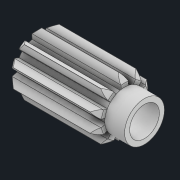
# Autodesk Inventor part: Steering Gear
Saved by Autodesk Inventor 2021 (Build 250183000, 183)
## iProperties
Created: 2020-10-15
Part Number: Steering Gear
Material: Generic
Document SubType Name: Modeling
Designer: Eugene Tang
Mass: 13.0101 g
Surface Area: 104.256 cm^2
Volume: 13.0101 cm^3
Density: 1 g/cm^3
Appearance: Default
ToothH: 5.620 mm
contact: 26.000 mm
rackteethprofileDepth: 2.411 mm
rackteethprofileLong: 3.683 mm
rackteethprofileShort: 2.480 mm
SteererGearPlane: 18.760 mm
GearLength: 45.000 mm
d1: 15.000 mm
Author: Eugene Tang
Autodesk Inventor part; units mm, degrees
ref_plane "YZ Plane" through (0, 0, 0) normal (1, 0, 0) x (0, 1, 0)
ref_plane "XZ Plane" through (0, 0, 0) normal (0, 1, 0) x (-1, 0, 0)
ref_plane "XY Plane" through (0, 0, 0) normal (0, 0, 1) x (1, 0, 0)
sketch "Sketch1" plane through (0, 0, 0) normal (1, 0, 0) x (0, 1, 0)
  circle A0 centre (0, 0) radius 11 construction
  circle A1 centre (0, 0) radius 7.5
  circle A2 centre (0, 0) radius 15
  line L0 (0, 0) -> (10.8109, -2.0308) construction
  line L1 (0, 0) -> (10.9093, 1.4093) construction
  line L2 (0, 0) -> (9.9399, 4.7115) construction
  line L3 (0, 0) -> (7.9975, 7.5525) construction
  line L4 (0, 0) -> (5.2722, 9.6542) construction
  line L5 (0, 0) -> (2.0308, 10.8109) construction
  line L6 (2.0308, 10.8109) -> (18.9428, 7.634) construction
  line L7 (5.2722, 9.6542) -> (17.3542, 3.0562) construction
  line L8 (7.9975, 7.5525) -> (15.0863, 0.0461) construction
  line L9 (9.9399, 4.7115) -> (12.8881, -1.5082) construction
  line L10 (10.9093, 1.4093) -> (10.8109, -2.0308) construction
  spline S0 degree 4 poles (10.8109, -2.0308) (13.448, -1.9078) (15.839, -0.0396) (18.3147, 3.5093) (18.9428, 7.634) knots 0 0 0 0 0 1 1 1 1 1 construction
  circle A3 centre (0, 0) radius 12 construction
  circle A4 centre (0, 0) radius 15.5 construction
  line L11 (0, 0) -> (15.3092, -2.4247) construction
  line L12 (-22.7177, 0) -> (27.8064, 0) construction
  circle A5 centre (0, 0) radius 9.38
  line L13 (11.8523, -1.8772) -> (-15, 0) construction
  circle A6 centre (0, 0) radius 13 construction
  dimension "d0" = 22
  dimension "d2" = 30
  dimension "d14" = 24
  dimension "d15" = 0.5
  dimension "d30" = 4
  dimension "d1" = 15
  dimension "angle" = 90
  dimension "d9" = 6.8831
  dimension "d10" = 10.3247
  dimension "d11" = 13.7662
  dimension "d13" = 17.2078
  dimension "d16" = 9
  dimension "SteererGearPlane" = 18.76
  dimension "ToothH" = 5.62
  dimension "d31" = 2
  dimension "contact" = 26
  constraints: 26 end point, 7 coincident, 3 centre point, 1 concentric, 1 horizontal alignment, 1 point on line, 39 other
  measures "d1" diameter of A1
  measures "d9" distance of L2.end L9.end
  measures "d10" distance of L3.end L8.end
  measures "d11" distance of L4.end L7.end
  measures "d13" distance of L5.end L6.end
  measures "d16" angle to the sketch x axis of L11
  measures "SteererGearPlane" diameter of A5
  measures "contact" diameter of A6
sketch "Sketch2" plane through (0, 0, 0) normal (1, 0, 0) x (0, 1, 0)
  circle A0 centre (0, 0) radius 12 construction
  line L0 (10.9093, 1.4093) -> (10.8109, -2.0308) construction
  line L1 (9.9399, 4.7115) -> (12.8881, -1.5082) construction
  line L2 (7.9975, 7.5525) -> (15.0863, 0.0461) construction
  line L3 (5.2722, 9.6542) -> (17.3542, 3.0562) construction
  line L4 (2.0308, 10.8109) -> (18.9428, 7.634) construction
  circle A1 centre (0, 0) radius 7.5 projected
  circle A2 centre (0, 0) radius 9.38 projected
  circle A3 centre (0, 0) radius 15 projected
  line L5 (11.8523, -1.8772) -> (-15, 0) construction
  spline S0 degree 4 poles (10.8109, -2.0308) (13.448, -1.9078) (15.839, -0.0396) (18.3147, 3.5093) (18.9428, 7.634) knots 0 0 0 0 0 1 1 1 1 1
  line L6 (11.8523, -1.8772) -> (9.2258, -1.6936)
  line L7 (-28.8241, 0) -> (28.8241, 0) construction
  spline S1 degree 4 poles (10.8109, 2.0308) (13.448, 1.9078) (15.839, 0.0396) (18.3147, -3.5093) (18.9428, -7.634) knots 0 0 0 0 0 1 1 1 1 1
  line L8 (11.8523, 1.8772) -> (9.2258, 1.6936)
  spline S2 degree 4 poles (9.9399, 4.7115) (12.0011, 6.3611) (12.8373, 9.2779) (12.7542, 13.6042) (10.8379, 17.3103) knots 0 0 0 0 0 1 1 1 1 1
  spline S3 degree 4 poles (7.5525, 7.9975) (9.7583, 9.448) (12.7908, 9.3419) (16.8796, 7.9261) (19.8122, 4.9583) knots 0 0 0 0 0 1 1 1 1 1
  line L9 (8.4853, 8.4853) -> (6.4684, 6.793)
  line L10 (10.6921, 5.4479) -> (8.4593, 4.0527)
  spline S4 degree 4 poles (5.2722, 9.6542) (5.9701, 12.2003) (4.9321, 15.0516) (2.3221, 18.5028) (-1.4067, 20.3747) knots 0 0 0 0 0 1 1 1 1 1
  spline S5 degree 4 poles (1.4093, 10.9093) (2.3413, 13.3794) (4.8569, 15.076) (8.9971, 16.3339) (13.114, 15.6566) knots 0 0 0 0 0 1 1 1 1 1
  line L11 (1.8772, 11.8523) -> (1.2402, 9.2976)
  line L12 (5.4479, 10.6921) -> (4.4617, 8.2509)
  spline S6 degree 4 poles (-1.4093, 10.9093) (-2.3413, 13.3794) (-4.8569, 15.076) (-8.9971, 16.3339) (-13.114, 15.6566) knots 0 0 0 0 0 1 1 1 1 1
  spline S7 degree 4 poles (-5.2722, 9.6542) (-5.9701, 12.2003) (-4.9321, 15.0516) (-2.3221, 18.5028) (1.4067, 20.3747) knots 0 0 0 0 0 1 1 1 1 1
  line L13 (-5.4479, 10.6921) -> (-4.4617, 8.2509)
  line L14 (-1.8772, 11.8523) -> (-1.2402, 9.2976)
  spline S8 degree 4 poles (-7.5525, 7.9975) (-9.7583, 9.448) (-12.7908, 9.3419) (-16.8796, 7.9261) (-19.8122, 4.9583) knots 0 0 0 0 0 1 1 1 1 1
  spline S9 degree 4 poles (-9.9399, 4.7115) (-12.0011, 6.3611) (-12.8373, 9.2779) (-12.7542, 13.6042) (-10.8379, 17.3103) knots 0 0 0 0 0 1 1 1 1 1
  line L15 (-10.6921, 5.4479) -> (-8.4593, 4.0527)
  line L16 (-8.4853, 8.4853) -> (-6.4684, 6.793)
  spline S10 degree 4 poles (-10.8109, 2.0308) (-13.448, 1.9078) (-15.839, 0.0396) (-18.3147, -3.5093) (-18.9428, -7.634) knots 0 0 0 0 0 1 1 1 1 1
  spline S11 degree 4 poles (-10.8109, -2.0308) (-13.448, -1.9078) (-15.839, -0.0396) (-18.3147, 3.5093) (-18.9428, 7.634) knots 0 0 0 0 0 1 1 1 1 1
  line L17 (-11.8523, -1.8772) -> (-9.2258, -1.6936)
  line L18 (-11.8523, 1.8772) -> (-9.2258, 1.6936)
  spline S12 degree 4 poles (-9.9399, -4.7115) (-12.0011, -6.3611) (-12.8373, -9.2779) (-12.7542, -13.6042) (-10.8379, -17.3103) knots 0 0 0 0 0 1 1 1 1 1
  spline S13 degree 4 poles (-7.5525, -7.9975) (-9.7583, -9.448) (-12.7908, -9.3419) (-16.8796, -7.9261) (-19.8122, -4.9583) knots 0 0 0 0 0 1 1 1 1 1
  line L19 (-8.4853, -8.4853) -> (-6.4684, -6.793)
  line L20 (-10.6921, -5.4479) -> (-8.4593, -4.0527)
  spline S14 degree 4 poles (-5.2722, -9.6542) (-5.9701, -12.2003) (-4.9321, -15.0516) (-2.3221, -18.5028) (1.4067, -20.3747) knots 0 0 0 0 0 1 1 1 1 1
  spline S15 degree 4 poles (-1.4093, -10.9093) (-2.3413, -13.3794) (-4.8569, -15.076) (-8.9971, -16.3339) (-13.114, -15.6566) knots 0 0 0 0 0 1 1 1 1 1
  line L21 (-1.8772, -11.8523) -> (-1.2402, -9.2976)
  line L22 (-5.4479, -10.6921) -> (-4.4617, -8.2509)
  spline S16 degree 4 poles (1.4093, -10.9093) (2.3413, -13.3794) (4.8569, -15.076) (8.9971, -16.3339) (13.114, -15.6566) knots 0 0 0 0 0 1 1 1 1 1
  spline S17 degree 4 poles (5.2722, -9.6542) (5.9701, -12.2003) (4.9321, -15.0516) (2.3221, -18.5028) (-1.4067, -20.3747) knots 0 0 0 0 0 1 1 1 1 1
  line L23 (5.4479, -10.6921) -> (4.4617, -8.2509)
  line L24 (1.8772, -11.8523) -> (1.2402, -9.2976)
  spline S18 degree 4 poles (7.5525, -7.9975) (9.7583, -9.448) (12.7908, -9.3419) (16.8796, -7.9261) (19.8122, -4.9583) knots 0 0 0 0 0 1 1 1 1 1
  spline S19 degree 4 poles (9.9399, -4.7115) (12.0011, -6.3611) (12.8373, -9.2779) (12.7542, -13.6042) (10.8379, -17.3103) knots 0 0 0 0 0 1 1 1 1 1
  line L25 (10.6921, -5.4479) -> (8.4593, -4.0527)
  line L26 (8.4853, -8.4853) -> (6.4684, -6.793)
  arc A4 (-9.2258, -1.6936) -> (-8.4593, -4.0527) centre (0, 0) ccw
  arc A5 (-6.4684, -6.793) -> (-4.4617, -8.2509) centre (0, 0) ccw
  arc A6 (-1.2402, -9.2976) -> (1.2402, -9.2976) centre (0, 0) ccw
  arc A7 (4.4617, -8.2509) -> (6.4684, -6.793) centre (0, 0) ccw
  arc A8 (8.4593, -4.0527) -> (9.2258, -1.6936) centre (0, 0) ccw
  arc A9 (9.2258, 1.6936) -> (8.4593, 4.0527) centre (0, 0) ccw
  arc A10 (6.4684, 6.793) -> (4.4617, 8.2509) centre (0, 0) ccw
  arc A11 (1.2402, 9.2976) -> (-1.2402, 9.2976) centre (0, 0) ccw
  arc A12 (-4.4617, 8.2509) -> (-6.4684, 6.793) centre (0, 0) ccw
  arc A13 (-8.4593, 4.0527) -> (-9.2258, 1.6936) centre (0, 0) ccw
  line L27 (1.2402, -9.2976) -> (-1.2402, -9.2976) construction
  line L28 (-0.4196, -9.2976) -> (-0.4196, -11.7086) construction
  line L29 (1.8414, -11.7086) -> (-1.8414, -11.7086) construction
  point P0 (12.8881, 1.5082)
  point P1 (15.0863, -0.0461)
  point P2 (17.3542, -3.0562)
  point P3 (12.178, 8.9048)
  point P4 (12.2434, 12.6731)
  point P5 (11.3132, 6.3552)
  point P6 (12.2322, 8.8303)
  point P7 (15.8363, 7.728)
  point P8 (9.5402, 8.7956)
  point P9 (4.6181, 14.3622)
  point P10 (2.4561, 17.4493)
  point P11 (5.4171, 11.7912)
  point P12 (4.7057, 14.3337)
  point P13 (8.2694, 15.5604)
  point P14 (2.5482, 12.7234)
  point P15 (-4.7057, 14.3337)
  point P16 (-8.2694, 15.5604)
  point P17 (-2.5482, 12.7234)
  point P18 (-4.6181, 14.3622)
  point P19 (-2.4561, 17.4493)
  point P20 (-5.4171, 11.7912)
  point P21 (-12.2322, 8.8303)
  point P22 (-15.8363, 7.728)
  point P23 (-9.5402, 8.7956)
  point P24 (-12.178, 8.9048)
  point P25 (-12.2434, 12.6731)
  point P26 (-11.3132, 6.3552)
  point P27 (-15.0863, -0.0461)
  point P28 (-17.3542, -3.0562)
  point P29 (-12.8881, 1.5082)
  point P30 (-15.0863, 0.0461)
  point P31 (-17.3542, 3.0562)
  point P32 (-12.8881, -1.5082)
  point P33 (-12.178, -8.9048)
  point P34 (-12.2434, -12.6731)
  point P35 (-11.3132, -6.3552)
  point P36 (-12.2322, -8.8303)
  point P37 (-15.8363, -7.728)
  point P38 (-9.5402, -8.7956)
  point P39 (-4.6181, -14.3622)
  point P40 (-2.4561, -17.4493)
  point P41 (-5.4171, -11.7912)
  point P42 (-4.7057, -14.3337)
  point P43 (-8.2694, -15.5604)
  point P44 (-2.5482, -12.7234)
  point P45 (4.7057, -14.3337)
  point P46 (8.2694, -15.5604)
  point P47 (2.5482, -12.7234)
  point P48 (4.6181, -14.3622)
  point P49 (2.4561, -17.4493)
  point P50 (5.4171, -11.7912)
  point P51 (12.2322, -8.8303)
  point P52 (15.8363, -7.728)
  point P53 (9.5402, -8.7956)
  point P54 (12.178, -8.9048)
  point P55 (12.2434, -12.6731)
  point P56 (11.3132, -6.3552)
  point P57 (12.1567, 8.7872)
  point P58 (12.1138, 8.8463)
  point P59 (4.6699, 14.2545)
  point P60 (4.6005, 14.2771)
  point P61 (-4.6005, 14.2771)
  point P62 (-4.6699, 14.2545)
  point P63 (-12.1138, 8.8463)
  point P64 (-12.1567, 8.7872)
  point P65 (-15, 0.0365)
  point P66 (-15, -0.0365)
  point P67 (-12.1567, -8.7872)
  point P68 (-12.1138, -8.8463)
  point P69 (-4.6699, -14.2545)
  point P70 (-4.6005, -14.2771)
  point P71 (4.6005, -14.2771)
  point P72 (4.6699, -14.2545)
  point P73 (12.1138, -8.8463)
  point P74 (12.1567, -8.7872)
  point P75 (15, -0.0365)
  point P76 (15, 0.0365)
  dimension "d20" = 360
  dimension "rackteethprofileDepth" = 2.411
  dimension "rackteethprofileLong" = 3.6828
  dimension "rackteethprofileShort" = 2.4805
  dimension "d36" = 1.4218
  constraints: 46 end point, 20 point on circle, 10 centre point, 7 symmetric about line, 5 point on line, 2 horizontal, 1 coincident, 1 perpendicular, 285 other
  measures "rackteethprofileDepth" distance of L28.start L28.end
  measures "rackteethprofileLong" distance of L29.start L29.end
  measures "rackteethprofileShort" distance of L24.end L21.end
  measures "d36" distance of L29.end L28.end
extrude "Extrusion1" add sketch "Sketch2" along normal blind 45 contours A2 | A2 L8 S1 A3 S0 L6 | A2 L9 S3 A3 S2 L10 | L25 S19 A3 S18 L26 A2 | A2 L11 S5 A3 S4 L12 | L23 S17 A3 S16 L24 A2 | A2 L13 S7 A3 S6 L14 | L21 S15 A3 S14 L22 A2 | A2 L15 S9 A3 S8 L16 | L19 S13 A3 S12 L20 A2 | A2 L17 S11 A3 S10 L18
sketch "Sketch3" plane through (0, 0, 0) normal (0, 0, 1) x (1, 0, 0)
  line L0 (0, 11.8523) -> (0, 15) projected
  line L1 (0, 15) -> (45, 15) projected
  line L2 (45, 11.8523) -> (45, 15) projected
  line L3 (0, 11.8523) -> (45, 11.8523) projected
  line L4 (0, 9.2258) -> (0, 11.8523) projected
  line L5 (0, 11.8523) -> (45, 11.8523) projected
  line L6 (45, 9.2258) -> (45, 11.8523) projected
  line L7 (0, 9.2258) -> (45, 9.2258) projected
  line L8 (0, 11.8523) -> (5, 16.8523)
  line L9 (5, 16.8523) -> (0, 16.8523)
  line L10 (0, -22.7177) -> (0, 27.8064) projected
  line L11 (45, 11.8523) -> (40, 16.8523)
  line L12 (40, 16.8523) -> (45, 16.8523)
  line L13 (45, 16.8523) -> (45, 15)
  line L14 (0, 0) -> (20.9473, 0) construction
  dimension "d24" = 45
  dimension "d25" = 5
  dimension "d26" = 5
  dimension "d27" = 45
  constraints: 12 end point, 3 horizontal, 1 perpendicular, 1 point on line
  measures "d24" angle of L0 L8
  measures "d25" distance of L8.end L9.end
  measures "d26" distance of L11.end L12.end
  measures "d27" angle of L13 L11
revolve "Revolution1" cut sketch "Sketch3" angle 360 about axis through (0, 0, 0) along (1, 0, 0) contours L0 L1 L8 | L10 L9 L8 L1 | L11 L1 L2 | L1 L11 L12 L13
sketch "Sketch4" plane through (45, 0, 0) normal (1, 0, 0) x (0, 0, -1)
  circle A0 centre (0, 0) radius 10.05
  circle A1 centre (0, 0) radius 7.5 projected
  dimension "d37" = 15
  dimension "d38" = 20.1
  constraints: 1 centre point, 1 coincident
  measures "d37" diameter of A1
  measures "d38" diameter of A0
extrude "Extrusion2" add sketch "Sketch4" along normal blind 10
equation "\"d9\" = 2 * d12"
equation "\"d10\" = 3 * d12"
equation "\"d11\" = 4 * d12"
equation "\"d13\" = 5 * d12"
equation "\"d31\" = 0.5 * d30"
equation "\"d22\" = GearLength"
equation "\"d26\" = d25"
equation "\"d27\" = d24"
equation "\"d38\" = 1.34 * d37"
equation "\"GearLength\" = 45"
equation "\"d12\" = 3.441558"
body "Solid1"
